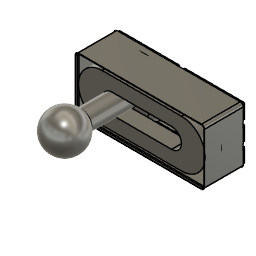
Joystick (Autodesk Fusion 360 design; units mm, degrees)
Autodesk Fusion 360 part; units mm, degrees
sketch "Sketch1" plane through (0, 0, 0) normal (0, 0, 1) x (1, 0, 0) in component "Component"
  line L0 (0, -30) -> (100, -30)
  arc A0 (100, -30) -> (100, 30) centre (100, 0) ccw
  line L1 (100, 30) -> (0, 30)
  arc A1 (0, 30) -> (0, -30) centre (0, 0) ccw
  line L2 (0, 0) -> (100, 0) construction
  dimension "d1" = 60
  constraint tangent L0 A0
  constraint tangent A0 L1
  constraint parallel L0 L1
  constraint tangent L1 A1
  constraint tangent L0 A1
  constraint horizontal L2
  constraint coincident A1.centre L2.start
  measures "d1" diameter of A0
extrude "Extrude1" add sketch "Sketch1" along normal blind 20 makes body 1 in component "Component"
sketch "Sketch2" plane through (0, 0, 0) normal (0, 0, 1) x (1, 0, 0) in component "Component"
  line L0 (12.5, -12.5) -> (87.5, -12.5)
  arc A0 (87.5, -12.5) -> (87.5, 12.5) centre (87.5, 0) ccw
  line L1 (87.5, 12.5) -> (12.5, 12.5)
  arc A1 (12.5, 12.5) -> (12.5, -12.5) centre (12.5, 0) ccw
  line L2 (0, 0) -> (100, 0) construction
  dimension "d4" = 25
  constraint tangent L0 A0
  constraint tangent A0 L1
  constraint parallel L0 L1
  constraint tangent L1 A1
  constraint tangent L0 A1
  constraint midpoint A1 L2.start
  constraint midpoint A0 L2.end
  constraint horizontal L2
  constraint coincident L2.start origin
  measures "d4" diameter of A0
extrude "Extrude2" cut sketch "Sketch2" along normal through all bodies 1 in component "Component"
sketch "Sketch3" plane through (0, 0, 0) normal (0, 0, 1) x (1, 0, 0) in component "Component"
sketch "Sketch1 (2)" plane through (0, 0, 0) normal (0, 0, 1) x (1, 0, 0) in component "Component'"
  circle A0 centre (-90, 0) radius 35
  dimension "d6" = 70
  measures "d6" diameter of A0
extrude "Extrude1'" add sketch "Sketch1 (2)" along normal blind 20 draft -20 separate body makes body 2 in component "Component'"
sketch "Sketch2 (2)" plane through (0, 0, 0) normal (0, 0, 1) x (1, 0, 0) in component "Component'"
  circle A0 centre (-90, 0) radius 12.5
  dimension "d10" = 25
  measures "d10" diameter of A0
extrude "Extrude2'" add sketch "Sketch2 (2)" along normal blind 80 bodies 2 in component "Component'"
extrude "Extrude3" add 1 faces at (-86.1912, -3.534, 80) along direction (0, 0, 1) blind 20 on bodies 2 bodies 2 in component "Component'"
sphere "SpherePrimitive1" add diameter 50 placed x (1, 0, 0) y (0, 1, 0) z (0, 0, 1) at (-90, 0, 100) bodies 2 in component "Component'"
ref_plane "WorkPlane1" through (0, 0, 0) normal (0, 0, 1) x (1, 0, 0) in component "Gridfinity bin 3x2x5"
sketch "Base plate sketch" plane through (0, 0, 0) normal (0, 0, 1) x (1, 0, 0) in component "Gridfinity bin 3x2x5"
  line L0 (-0.25, -0.25) -> (81.75, -0.25)
  line L1 (81.75, -0.25) -> (81.75, 23.75)
  line L2 (81.75, 23.75) -> (-0.25, 23.75)
  line L3 (-0.25, 23.75) -> (-0.25, -0.25)
  dimension "d26" = 0.25
  dimension "d27" = 0.25
  dimension "d28" = 82
  dimension "d29" = 24
  constraint horizontal L0
  constraint vertical L1
  constraint horizontal L2
  constraint vertical L3
  measures "d26" vertical distance of origin L0.start
  measures "d27" horizontal distance of origin L2.end
  measures "d28" horizontal distance of L0.start L0.end
  measures "d29" vertical distance of L0.end L1.end
extrude "Base top section extrude" add sketch "Base plate sketch" against normal blind 2.4 separate body makes body 3 in component "Gridfinity bin 3x2x5"
fillet "Base corner fillet" radius 4 8 edges at (-0.25, -0.25, -1.2) (81.75, -0.25, -1.2) (81.75, -0.25, -1.2) (81.75, 23.75, -1.2) (81.75, 23.75, -1.2) (-0.25, 23.75, -1.2) (-0.25, 23.75, -1.2) (-0.25, -0.25, -1.2) on bodies 3 in component "Gridfinity bin 3x2x5"
chamfer "Chamfer1" distance 2.4 angle 45 8 edges at (0.9216, 22.5784, -2.4) (-0.25, 11.75, -2.4) (0.9216, 0.9216, -2.4) (40.75, -0.25, -2.4) (80.5784, 0.9216, -2.4) (81.75, 11.75, -2.4) (80.5784, 22.5784, -2.4) (40.75, 23.75, -2.4) on bodies 3 in component "Gridfinity bin 3x2x5"
extrude "Extrude2''" add 1 faces at (53.0833, 8.5498, -2.4) along direction (0, 0, -1) blind 2.6 on bodies 3 bodies 3 in component "Gridfinity bin 3x2x5"
chamfer "Chamfer2" distance 0.8 angle 45 8 edges at (2.6186, 20.8814, -5) (40.75, 21.35, -5) (78.8814, 20.8814, -5) (79.35, 11.75, -5) (78.8814, 2.6186, -5) (40.75, 2.15, -5) (2.6186, 2.6186, -5) (2.15, 11.75, -5) on bodies 3 in component "Gridfinity bin 3x2x5"
pattern_linear "R-Pattern1" count 2 spacing 82 along (1, 0, 0) count 3 spacing 24 along (0, 1, 0) of bodies 3 makes body 4 at (135.0833, 7.75, 0) makes body 5 at (53.0833, 31.75, 0) makes body 6 at (135.0833, 31.75, 0) makes body 7 at (53.0833, 55.75, 0) makes body 8 at (135.0833, 55.75, 0) in component "Gridfinity bin 3x2x5"
sketch "Simple box sketch" plane through (0, 0, 0) normal (0, 0, 1) x (1, 0, 0) in component "Gridfinity bin 3x2x5"
  line L0 (0, 0) -> (163.5, 0)
  line L1 (163.5, 0) -> (163.5, 71.5)
  line L2 (163.5, 71.5) -> (0, 71.5)
  line L3 (0, 71.5) -> (0, 0)
  dimension "d42" = 163.5
  dimension "d43" = 71.5
  constraint horizontal L0
  constraint vertical L1
  constraint horizontal L2
  constraint vertical L3
  constraint coincident L0.start L3
  constraint coincident L3.end L0
  measures "d42" horizontal distance of L0.start L0.end
  measures "d43" vertical distance of L0.end L1.end
extrude "Simple box extrude" add sketch "Simple box sketch" along normal blind 45 separate body makes body 9 in component "Gridfinity bin 3x2x5"
fillet "Bin body corner fillets" radius 3.75 8 edges at (0, 71.5, 22.5) (163.5, 71.5, 22.5) (0, 0, 22.5) (0, 71.5, 22.5) (163.5, 71.5, 22.5) (163.5, 0, 22.5) (163.5, 0, 22.5) (0, 0, 22.5) on bodies 9 in component "Gridfinity bin 3x2x5"
ref_plane "WorkPlane2" through (0, 0, 45) normal (0, 0, 1) x (1, 0, 0) in component "Gridfinity bin 3x2x5"
sketch "Simple box at point sketch" plane through (0, 0, 45) normal (0, 0, 1) x (1, 0, 0) in component "Gridfinity bin 3x2x5"
  line L0 (0, 0) -> (163.5, 0)
  line L1 (163.5, 0) -> (163.5, 71.5)
  line L2 (163.5, 71.5) -> (0, 71.5)
  line L3 (0, 71.5) -> (0, 0)
  dimension "d49" = 163.5
  dimension "d50" = 71.5
  constraint horizontal L0
  constraint vertical L1
  constraint horizontal L2
  constraint vertical L3
  constraint coincident L0.start L3
  constraint coincident L3.end L0
  measures "d49" horizontal distance of L0.start L0.end
  measures "d50" vertical distance of L0.end L1.end
extrude "Simple box at point extrude" add sketch "Simple box at point sketch" along normal blind 4.4 separate body makes body 10 in component "Gridfinity bin 3x2x5"
fillet "Lip body corner fillets" radius 3.75 8 edges at (0, 71.5, 47.2) (163.5, 71.5, 47.2) (0, 0, 47.2) (0, 71.5, 47.2) (163.5, 71.5, 47.2) (163.5, 0, 47.2) (163.5, 0, 47.2) (0, 0, 47.2) on bodies 10 in component "Gridfinity bin 3x2x5"
ref_plane "WorkPlane3" through (0, 0, 50) normal (0, 0, 1) x (1, 0, 0) in component "Gridfinity bin 3x2x5"
sketch "Base plate sketch (1)" plane through (0, 0, 50) normal (0, 0, 1) x (1, 0, 0) in component "Gridfinity bin 3x2x5"
  line L0 (-0.5, -0.5) -> (164, -0.5)
  line L1 (164, -0.5) -> (164, 72)
  line L2 (164, 72) -> (-0.5, 72)
  line L3 (-0.5, 72) -> (-0.5, -0.5)
  dimension "d56" = 0.5
  dimension "d57" = 0.5
  dimension "d58" = 164.5
  dimension "d59" = 72.5
  constraint horizontal L0
  constraint vertical L1
  constraint horizontal L2
  constraint vertical L3
  measures "d56" vertical distance of origin L0.start
  measures "d57" horizontal distance of origin L2.end
  measures "d58" horizontal distance of L0.start L0.end
  measures "d59" vertical distance of L0.end L1.end
extrude "Base top section extrude (1)" add sketch "Base plate sketch (1)" against normal blind 2.4 separate body makes body 11 in component "Gridfinity bin 3x2x5"
fillet "Base corner fillet (1)" radius 4.25 8 edges at (-0.5, -0.5, 48.8) (164, -0.5, 48.8) (164, -0.5, 48.8) (164, 72, 48.8) (164, 72, 48.8) (-0.5, 72, 48.8) (-0.5, 72, 48.8) (-0.5, -0.5, 48.8) on bodies 11 in component "Gridfinity bin 3x2x5"
chamfer "Chamfer3" distance 2.4 angle 45 8 edges at (0.7448, 70.7552, 47.6) (-0.5, 35.75, 47.6) (0.7448, 0.7448, 47.6) (81.75, -0.5, 47.6) (162.7552, 0.7448, 47.6) (164, 35.75, 47.6) (162.7552, 70.7552, 47.6) (81.75, 72, 47.6) on bodies 11 in component "Gridfinity bin 3x2x5"
extrude "Extrude6" add 1 faces at (107.75, 24.4665, 47.6) along direction (0, 0, -1) blind 2.6 on bodies 11 bodies 11 in component "Gridfinity bin 3x2x5"
ref_plane "WorkPlane4" through (81.75, 35.75, 49.4) normal (0, 0, 1) x (1, 0, 0) in component "Gridfinity bin 3x2x5"
sketch "Lip top chamfer" plane through (0, 0, 49.4) normal (0, 0, 1) x (1, 0, 0) in component "Gridfinity bin 3x2x5"
  line L0 (0, 0) -> (163.5, 0)
  line L1 (163.5, 0) -> (163.5, 71.5)
  line L2 (163.5, 71.5) -> (0, 71.5)
  line L3 (0, 71.5) -> (0, 0)
  dimension "d68" = 163.5
  dimension "d69" = 71.5
  constraint horizontal L0
  constraint vertical L1
  constraint horizontal L2
  constraint vertical L3
  constraint coincident L0.start L3
  constraint coincident L3.end L0
  measures "d68" horizontal distance of L0.start L0.end
  measures "d69" vertical distance of L0.end L1.end
extrude "Lip top chamfer cut" add sketch "Lip top chamfer" against normal blind 0.6 separate body makes body 12 in component "Gridfinity bin 3x2x5"
combine "Combine1" operation cut target body 10 tool bodies 12 11 in component "Gridfinity bin 3x2x5"
ref_plane "WorkPlane5" through (0, 0, 45) normal (0, 0, 1) x (1, 0, 0) in component "Gridfinity bin 3x2x5"
sketch "Simple box at point sketch (1)" plane through (0, 0, 45) normal (0, 0, 1) x (1, 0, 0) in component "Gridfinity bin 3x2x5"
  line L0 (1.2, 1.2) -> (162.3, 1.2)
  line L1 (162.3, 1.2) -> (162.3, 70.3)
  line L2 (162.3, 70.3) -> (1.2, 70.3)
  line L3 (1.2, 70.3) -> (1.2, 1.2)
  dimension "d73" = 1.2
  dimension "d74" = 1.2
  dimension "d75" = 161.1
  dimension "d76" = 69.1
  constraint horizontal L0
  constraint vertical L1
  constraint horizontal L2
  constraint vertical L3
  measures "d73" vertical distance of origin L0.start
  measures "d74" horizontal distance of origin L2.end
  measures "d75" horizontal distance of L0.start L0.end
  measures "d76" vertical distance of L0.end L1.end
extrude "Lip bottom chamfer extrude" add sketch "Simple box at point sketch (1)" along normal blind 2.55 separate body makes body 13 in component "Gridfinity bin 3x2x5"
fillet "Fillet5" radius 2.55 8 edges at (1.2, 70.3, 46.275) (162.3, 70.3, 46.275) (1.2, 1.2, 46.275) (1.2, 70.3, 46.275) (162.3, 70.3, 46.275) (162.3, 1.2, 46.275) (162.3, 1.2, 46.275) (1.2, 1.2, 46.275) on bodies 13 in component "Gridfinity bin 3x2x5"
chamfer "Chamfer4" distance 2.55 angle 45 8 edges at (1.9469, 1.9469, 47.55) (81.75, 1.2, 47.55) (161.5531, 1.9469, 47.55) (162.3, 35.75, 47.55) (161.5531, 69.5531, 47.55) (81.75, 70.3, 47.55) (1.9469, 69.5531, 47.55) (1.2, 35.75, 47.55) on bodies 13 in component "Gridfinity bin 3x2x5"
combine "Combine2" operation cut target body 10 tool bodies 13 in component "Gridfinity bin 3x2x5"
ref_plane "WorkPlane6" through (0, 0, 45) normal (0, 0, 1) x (1, 0, 0) in component "Gridfinity bin 3x2x5"
sketch "Inner cutout sketch" plane through (0, 0, 45) normal (0, 0, 1) x (1, 0, 0) in component "Gridfinity bin 3x2x5"
  line L0 (1.2, 1.2) -> (162.3, 1.2)
  line L1 (162.3, 1.2) -> (162.3, 70.3)
  line L2 (162.3, 70.3) -> (1.2, 70.3)
  line L3 (1.2, 70.3) -> (1.2, 1.2)
  dimension "d83" = 1.2
  dimension "d84" = 1.2
  dimension "d85" = 161.1
  dimension "d86" = 69.1
  constraint horizontal L0
  constraint vertical L1
  constraint horizontal L2
  constraint vertical L3
  measures "d83" vertical distance of origin L0.start
  measures "d84" horizontal distance of origin L2.end
  measures "d85" horizontal distance of L0.start L0.end
  measures "d86" vertical distance of L0.end L1.end
extrude "Inner cutout extrude" add sketch "Inner cutout sketch" against normal blind 44 separate body makes body 14 in component "Gridfinity bin 3x2x5"
fillet "Fillet6" radius 2.55 8 edges at (1.2, 1.2, 23) (162.3, 1.2, 23) (162.3, 1.2, 23) (162.3, 70.3, 23) (162.3, 70.3, 23) (1.2, 70.3, 23) (1.2, 70.3, 23) (1.2, 1.2, 23) on bodies 14 in component "Gridfinity bin 3x2x5"
fillet "Fillet7" radius 2.55 8 edges at (81.75, 70.3, 1) (161.5531, 69.5531, 1) (162.3, 35.75, 1) (161.5531, 1.9469, 1) (81.75, 1.2, 1) (1.9469, 1.9469, 1) (1.2, 35.75, 1) (1.9469, 69.5531, 1) on bodies 14 in component "Gridfinity bin 3x2x5"
combine "Combine3" operation cut target body 9 tool bodies 14 in component "Gridfinity bin 3x2x5"
combine "Combine4" operation add target body 9 tool bodies 10 in component "Gridfinity bin 3x2x5"
ref_plane "WorkPlane7" through (0, 0, 0) normal (0, 0, 1) x (1, 0, 0) in component "Gridfinity bin 3x2x5"
sketch "Base clearance cut sketch" plane through (0, 0, 0) normal (0, 0, 1) x (1, 0, 0) in component "Gridfinity bin 3x2x5"
  line L0 (3.75, 0) -> (159.75, 0)
  line L1 (163.5, 3.75) -> (163.5, 67.75)
  line L2 (159.75, 71.5) -> (3.75, 71.5)
  line L3 (0, 67.75) -> (0, 3.75)
  arc A0 (159.75, 0) -> (163.5, 3.75) centre (159.75, 3.75) ccw
  arc A1 (163.5, 67.75) -> (159.75, 71.5) centre (159.75, 67.75) ccw
  arc A2 (3.75, 71.5) -> (0, 67.75) centre (3.75, 67.75) ccw
  arc A3 (0, 3.75) -> (3.75, 0) centre (3.75, 3.75) ccw
  arc A4 (159.75, -10) -> (173.5, 3.75) centre (159.75, 3.75) ccw
  line L4 (173.5, 3.75) -> (173.5, 67.75)
  arc A5 (173.5, 67.75) -> (159.75, 81.5) centre (159.75, 67.75) ccw
  line L5 (159.75, 81.5) -> (3.75, 81.5)
  arc A6 (3.75, 81.5) -> (-10, 67.75) centre (3.75, 67.75) ccw
  line L6 (-10, 67.75) -> (-10, 3.75)
  arc A7 (-10, 3.75) -> (3.75, -10) centre (3.75, 3.75) ccw
  line L7 (3.75, -10) -> (159.75, -10)
  point P0 (163.5, 0)
  point P1 (163.5, 71.5)
  dimension "d94" = 163.5
  dimension "d95" = 71.5
  dimension "d96" = 3.75
  dimension "d97" = 10
  constraint horizontal L0
  constraint vertical L1
  constraint horizontal L2
  constraint vertical L3
  constraint coincident origin L3
  constraint coincident origin L0
  constraint coincident P0 L0
  constraint coincident P0 L1
  constraint tangent L0 A0
  constraint tangent L1 A0
  constraint coincident P1 L1
  constraint coincident P1 L2
  constraint tangent L1 A1
  constraint tangent L2 A1
  constraint tangent L2 A2
  constraint tangent L3 A2
  constraint tangent L3 A3
  constraint tangent L0 A3
  constraint equal A0 A1
  constraint equal A1 A2
  constraint equal A2 A3
  measures "d94" horizontal distance of origin P0
  measures "d95" vertical distance of P0 P1
  measures "d96" radius of A0
extrude "Base side clearance cut" cut sketch "Base clearance cut sketch" along normal blind 1000 and the other way blind 1000 bodies 3 4 5 6 7 8 9 in component "Gridfinity bin 3x2x5"
combine "Combine5" operation add target body 9 tool bodies 4 5 6 7 8 3 3 in component "Gridfinity bin 3x2x5"
component "Component" placed x (1, 0, 0) y (0, 1, 0) z (0, 0, 1) at (0, 0, 0)
component "Component'" placed x (1, 0, 0) y (0, 1, 0) z (0, 0, 1) at (102.5, 0, -20)
component "Gridfinity bin 3x2x5" placed x (1, 0, 0) y (0, 1, 0) z (0, 0, 1) at (-32.9148, -36.0803, -27.3119)
equation "d1 = Length * 0.6"
equation "d2 = Length * 0.2"
equation "d4 = Length * 0.25"
equation "d6 = 1.4 * Radius"
equation "d7 = Height * 0.25"
equation "d10 = Length * 0.25"
equation "d11 = Height"
equation "d13 = Length * 0.2"
equation "d15 = Radius"
equation "Length = 100 mm"
equation "Radius = 50 mm"
equation "Height = 80 mm"
equation "d30 = -( 2.40 mm )"
equation "d60 = -( 2.40 mm )"
equation "d70 = -( 0.60 mm )"
equation "d87 = -( 44.00 mm )"
named bodies: "Base", "Base (1)", "Base (2)", "Base (3)", "Base (4)", "Base (5)", "Gridfinity bin 3x2x5", "Lip body", "Lip cutout", "Inner cutout"
